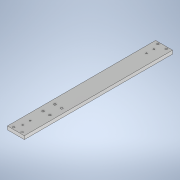
# Autodesk Inventor part: Lateral
Saved by Autodesk Inventor 2020 (Build 240168000, 168)
## iProperties
Created: 2020-05-08
Part Number: Lateral
Material: Aluminio 6061
Document SubType Name: Modeling
Designer: Pipi
Density: 2.7 g/cm^3
Appearance: Aluminum - Dark
Mass: 576.089 g
Surface Area: 535.299 cm^2
Volume: 213.366 cm^3
Author: Pipi
Autodesk Inventor part; units mm, degrees
ref_plane "YZ Plane" through (0, 0, 0) normal (1, 0, 0) x (0, 1, 0)
ref_plane "XZ Plane" through (0, 0, 0) normal (0, 1, 0) x (-1, 0, 0)
ref_plane "XY Plane" through (0, 0, 0) normal (0, 0, 1) x (1, 0, 0)
sketch "Boceto1" plane through (0, 0, 0) normal (0, 1, 0) x (-1, 0, 0)
  line L0 (14211.5164, 17617.1084) -> (14161.5164, 17617.1084)
  line L1 (14161.5164, 17617.1084) -> (14161.5164, 17179.1084)
  line L2 (14161.5164, 17179.1084) -> (14211.5164, 17179.1084)
  line L3 (14211.5164, 17179.1084) -> (14211.5164, 17617.1084)
  circle A0 centre (14191.5164, 17592.1084) radius 2
  circle A1 centre (14191.5164, 17570.1084) radius 2
  line L4 (14161.5164, 17398.1084) -> (14184, 17398.1084)
  circle A2 centre (14191.5164, 17204.1084) radius 2
  circle A3 centre (14191.5164, 17226.1084) radius 2
  dimension "d4" = 438
  dimension "d5" = 50
  dimension "d16" = 4
  dimension "d17" = 4
  dimension "d18" = 25
  dimension "d19" = 22
  dimension "d20" = 30
  dimension "d21" = 30
  constraints: 10 end point, 4 centre point, 3 perpendicular, 2 horizontal, 2 symmetric about line, 1 midpoint, 2 other
  measures "d4" distance of L0.end L1.end
  measures "d5" distance of L0.start L0.end
  measures "d16" diameter of A0
  measures "d17" diameter of A1
  measures "d18" distance from line of L0 A0.centre
  measures "d19" distance of A0.centre A1.centre
  measures "d20" distance from line of L1 A0.centre
  measures "d21" distance from line of L1 A1.centre
extrude "Extrusión1" add sketch "Boceto1" along normal blind 10
sketch "Boceto2" plane through (0, 10, 0) normal (0, 1, 0) x (1, 0, 0)
  line L0 (-14211.5164, -17617.1084) -> (-14161.5164, -17617.1084) projected
  line L1 (-14211.5164, -17617.1084) -> (-14211.5164, -17611.1084)
  line L2 (-14211.5164, -17179.1084) -> (-14211.5164, -17617.1084) projected
  line L3 (-14211.5164, -17611.1084) -> (-14161.5164, -17611.1084)
  line L4 (-14161.5164, -17617.1084) -> (-14161.5164, -17179.1084) projected
  line L5 (-14161.5164, -17179.1084) -> (-14211.5164, -17179.1084) projected
  line L6 (-14211.5164, -17179.1084) -> (-14211.5164, -17185.1084)
  line L7 (-14211.5164, -17185.1084) -> (-14161.5164, -17185.1084)
  line L8 (-14211.5164, -17611.1084) -> (-14199.0164, -17611.1084)
  line L9 (-14161.5164, -17185.1084) -> (-14174.0164, -17185.1084)
  circle A0 centre (-14199.0164, -17611.1084) radius 3
  circle A1 centre (-14174.0164, -17611.1084) radius 3
  circle A2 centre (-14199.0164, -17185.1084) radius 3
  circle A3 centre (-14174.0164, -17185.1084) radius 3
  dimension "d6" = 6
  dimension "d7" = 6
  dimension "d8" = 12.5
  dimension "d9" = 12.5
  dimension "d10" = 6
  dimension "d11" = 6
  dimension "d12" = 6
  dimension "d13" = 6
  dimension "d30" = 6
  constraints: 12 end point, 5 point on line, 4 centre point, 2 coincident, 2 perpendicular
  measures "d6" distance of L0.start L1.end
  measures "d7" distance of L2.start L6.end
  measures "d8" distance of L1.end L8.end
  measures "d9" distance of L7.end L9.end
  measures "d10" diameter of A0
  measures "d11" diameter of A1
  measures "d12" diameter of A2
  measures "d13" diameter of A3
  measures "d30" distance from line of L0 A1.centre
extrude "Extrusión2" cut sketch "Boceto2" against normal blind 20 contours A0 L3 | L3 A0 | A1 L3 | L3 A1 | A2 L7 | L7 A2 | A3 L7 | L7 A3
thread "Thread1" size "M4x0.7" class "6H" standard "ANSI Metric M Profile" length 40
thread "Thread2" size "M4x0.7" class "6H" standard "ANSI Metric M Profile" length 40
thread "Thread3" size "M4x0.7" class "6H" standard "ANSI Metric M Profile" length 40
thread "Thread4" size "M4x0.7" class "6H" standard "ANSI Metric M Profile" length 40
sketch "Boceto3" plane through (0, 0, 0) normal (0, -1, 0) x (1, 0, 0)
  line L0 (-14161.5164, 17617.1084) -> (-14161.5164, 17179.1084) projected
  line L1 (-14176.5164, 17526.8384) -> (-14196.5164, 17526.8384)
  line L2 (-14196.5164, 17526.8384) -> (-14196.5164, 17491.8384)
  line L3 (-14196.5164, 17491.8384) -> (-14176.5164, 17491.8384)
  line L4 (-14176.5164, 17491.8384) -> (-14176.5164, 17526.8384)
  circle A0 centre (-14176.5164, 17491.8384) radius 3
  circle A1 centre (-14196.5164, 17491.8384) radius 3
  circle A2 centre (-14176.5164, 17526.8384) radius 3
  circle A3 centre (-14196.5164, 17526.8384) radius 3
  line L5 (-14211.5164, 17617.1084) -> (-14161.5164, 17617.1084) projected
  line L6 (-14211.5164, 17179.1084) -> (-14211.5164, 17617.1084) projected
  dimension "d58" = 35
  dimension "d59" = 15
  dimension "d60" = 90.27
  dimension "d61" = 15
  dimension "d62" = 20
  constraints: 8 end point, 4 centre point, 4 coincident
  measures "d58" distance of L3.end L1.start
  measures "d59" distance between parallel lines of L0 L4
  measures "d60" distance between parallel lines of L5 L1
  measures "d61" distance between parallel lines of L6 L2
  measures "d62" distance between parallel lines of L2 L4
hole "Agujero1" at (-14176.5164, 0, 17526.8384) at (-14196.5164, 0, 17526.8384) at (-14176.5164, 0, 17491.8384) at (-14196.5164, 0, 17491.8384) direction (0, 1, 0) diameter 6 depth 12 tip angle 118
